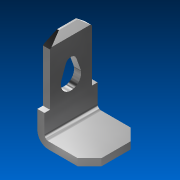
# Autodesk Inventor part: Soanar Power Module Pin C
Saved by Autodesk Inventor 2016 (Build 200138000, 138)
## iProperties
Created: 2013-08-06
Material: Nickel-Copper Alloy 400
Document SubType Name: Modeling
Designer: sdarley
Density: 8.83 g/cm^3
Appearance: Chrome - Polished
Project: Power Entry Module - Soanar PP4003
Description: Soanar Power Module Pin C
Author: sdarley
Title: Soanar Power Module Pin C
Revision Number: 1
Autodesk Inventor part; units mm, degrees
ref_plane "YZ Plane" through (0, 0, 0) normal (1, 0, 0) x (0, 1, 0)
ref_plane "XZ Plane" through (0, 0, 0) normal (0, 1, 0) x (-1, 0, 0)
ref_plane "XY Plane" through (0, 0, 0) normal (0, 0, 1) x (1, 0, 0)
sketch "Sketch1" plane through (0, 0, 0) normal (0, 1, 0) x (-1, 0, 0)
  line L0 (-5.9, 0) -> (-1.25, 0)
  line L1 (-5.9, 0) -> (-5.9, 0.8)
  line L2 (-5.9, 0.8) -> (-1.25, 0.8)
  line L3 (0, 1.25) -> (0, 10.35)
  line L4 (0, 10.35) -> (-0.8, 10.35)
  line L5 (-0.8, 10.35) -> (-0.8, 1.25)
  arc A0 (-1.25, 0) -> (0, 1.25) centre (-1.25, 1.25) ccw
  arc A1 (-1.25, 0.8) -> (-0.8, 1.25) centre (-1.25, 1.25) ccw
  point P0 (0, 0)
  dimension "d0" = 0.8
  dimension "d1" = 10.35
  dimension "d2" = 5.9
  dimension "d3" = 1.25
  constraints: 12 end point, 5 perpendicular, 4 point on circle, 4 tangent, 2 centre point, 1 concentric, 1 horizontal, 1 horizontal alignment, 1 parallel, 1 vertical alignment
  measures "d0" distance between parallel lines of L3 L5
  measures "d1" distance between parallel lines of L0 L4
  measures "d2" distance between parallel lines of L1 L3
  measures "d3" radius of A0
extrude "Extrusion1" add sketch "Sketch1" along normal mid plane 6
sketch "Sketch2" plane through (0.8, -3, 1.25) normal (1, 0, 0) x (0, 0, -1)
  line L0 (-9.1, 0) -> (-9.1, 6) projected
  arc A0 (-4.3396, 1.918) -> (-4.3396, 4.082) centre (-3.95, 3) ccw
  arc A1 (-5.6783, 3.6) -> (-5.6783, 2.4) centre (-5.4623, 3) ccw
  line L1 (-5.6783, 3.6) -> (-4.3396, 4.082)
  line L2 (-5.6783, 2.4) -> (-4.3396, 1.918)
  line L3 (1.25, 6) -> (1.25, 0) projected
  line L4 (-9.1, 6) -> (-2.1, 6)
  line L5 (-2.1, 6) -> (-2.1, 5.375)
  line L6 (-2.1, 5.375) -> (-9.1, 5.375)
  line L7 (-9.1, 5.375) -> (-9.1, 6)
  line L8 (-9.1, 0) -> (-2.1, 0)
  line L9 (-2.1, 0) -> (-2.1, 0.625)
  line L10 (-2.1, 0.625) -> (-9.1, 0.625)
  line L11 (-9.1, 0.625) -> (-9.1, 0)
  point P0 (1.25, 3)
  point P1 (1.25, 3)
  dimension "d6" = 3
  dimension "d7" = 3.3
  dimension "d8" = 1.15
  dimension "d9" = 1.2
  dimension "d27" = 4.75
  dimension "d28" = 7
  constraints: 20 end point, 4 parallel, 4 point on circle, 4 tangent, 2 centre point, 2 horizontal, 2 horizontal alignment, 2 perpendicular, 1 collinear, 1 midpoint, 1 vertical alignment
  measures "d6" distance edge to line of A1 L0
  measures "d8" radius of A0
  measures "d9" distance of L2.start L1.start
  measures "d27" distance between parallel lines of L10 L6
  measures "d28" distance between parallel lines of L5 L0
extrude "Extrusion2" cut sketch "Sketch2" against normal through all
chamfer "Chamfer1" distance 1.35 angle 45 2 edges at (5.9, 3, 0.4) (5.9, -3, 0.4)
chamfer "Chamfer2" distance 1.3 distance2 1.1 1 edges at (0.4, -2.375, 10.35) measured on face at (0.2667, -0.7917, 10.35)
chamfer "Chamfer3" distance 1.3 distance2 1.1 1 edges at (0.4, 2.375, 10.35) measured on face at (0.2667, 0.075, 10.35)
chamfer "Chamfer4" distance 0.3 distance2 0.95 1 edges at (0.8, 0, 10.35) measured on face at (0.2667, -0.3583, 10.35)
chamfer "Chamfer5" distance 0.3 distance2 0.95 1 edges at (0, 0, 10.35) measured on face at (0.1667, -0.3583, 10.35)
body "Solid1"
